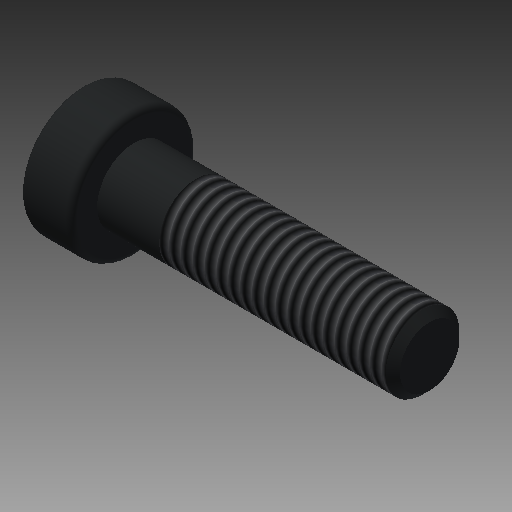
# Autodesk Inventor part: DIN-6912 - M5x20(F)
Saved by Autodesk Inventor 2017 (Build 210142000, 142)
## iProperties
Category: PARTsolutions
Company: FESTO
Created: 2018-05-29
Part Number: DIN-6912 - M5x20(F)
Catalog Web Link: www.cadenas.de
Description: DIN-6912-Hexagon socket head cap screw with centre hole and low head
Vendor: FESTO
Document SubType Name: Modeling
Designer: psAdmin
Manufacturer: FESTO
Mass: 0.545165 g
Surface Area: 5.48093 cm^2
Volume: 0.545165 cm^3
Density: 1 g/cm^3
Material: Generic
Appearance: PSOLRGB-46-51-51
PSOL_IDENT_0: {$CADENAS_DATA\23d-libs\festo\zyl_zubeh\din_6912\din_6912.prj},183 {VTYP=3D},{NB=DIN-6912 - M5x20(F)
PSOL_IDENT_1: },{LINA=DIN-6912 - M5x20(F)},{NN=DIN-6912},{DATE=16.11.2017 11:29:57},{GEOMDATE=16.11.2017 11:29:44}
PSOL_IDENT_2: ,{VERSION=},{LINEID=130},{LINESUBID=-1},{WBVAR=}  {NB=DIN-6912 - M5x20(F)},{LINA=DIN-6912 - M5x20(F)
PSOL_IDENT_3: },{KT=L},{IDNR=},{NENN=M5x20},{D=5.000},{L=20.000},{DK=4.019},{LS=1.800},{LG=4.200},{DK1=8.500},{DH=
PSOL_IDENT_4: 2.500},{K=3.500},{R=0.200},{V=0.400},{S=4.000},{T1=2.000},{T2=4.000},{F=0.600},{DA=5.700},{DW=7.700}
NN: DIN-6912
NT: Hexagon socket head cap screw with centre hole and low head
NB: DIN-6912 - M5x20(F)
NBSYN: DIN-6912 - $NENN.(F)
LINA: DIN-6912 - M5x20(F)
ROWDESC: M5x20
D: 5.000
L: 20.000
DK: 4.019
LS: 1.800
LG: 4.200
DK1: 8.500
DH: 2.500
K: 3.500
R: 0.200
V: 0.400
S: 4.000
T1: 2.000
T2: 4.000
F: 0.600
DA: 5.700
DW: 7.700
SUPPLIER: FESTO
ARTICLENO: DIN-6912 - M5x20(F)
BOMINFO: DIN-6912 - M5x20(F)
CREATOR: CADENAS GmbH
Title: DIN-6912 - M5x20(F)
Author: Cadenas PARTsolutions
Comments: Hexagon socket head cap screw with centre hole and low head
Autodesk Inventor part; units mm, degrees
sketch "Sketch_1" plane through (0, 0, 0) normal (0, 0, 1) x (1, 0, 0)
  line L0 (20, 0) -> (1.75, 0)
  line L1 (1.75, 0) -> (0.5, 1.25)
  line L2 (0.5, 1.25) -> (-0.75, 1.25)
  line L3 (-0.75, 1.25) -> (-1.5, 2)
  line L4 (-1.5, 2) -> (-3.1906, 2)
  line L5 (-3.1906, 2) -> (-3.5, 2.3094)
  line L6 (-3.5, 2.3094) -> (-3.5, 3.85)
  arc A0 (-3.1, 4.25) -> (-3.5, 3.85) centre (-3.1, 3.85) ccw
  line L7 (-3.1, 4.25) -> (-0.4, 4.25)
  arc A1 (0, 3.85) -> (-0.4, 4.25) centre (-0.4, 3.85) ccw
  line L8 (0, 3.85) -> (0, 2.5)
  line L9 (0, 2.5) -> (19.5095, 2.5)
  line L10 (19.5095, 2.5) -> (20, 2.0095)
  line L11 (20, 2.0095) -> (20, 0)
  line L12 (20, 0) -> (1.75, 0)
  constraints: 26 end point, 4 point on circle, 2 centre point
revolve "Revolution1" add sketch "Sketch_1" angle 360 about axis through (20, 0, 0) along (-1, 0, 0)
thread "Thread1" size "M5x0.8" class "6g" standard "ISO Metric profile" length 15.3095
sketch "Sketch_2" plane through (-3.5, 0, 0) normal (1, 0, 0) x (0, 0, -1)
  line L0 (-2, -1.1547) -> (0, -2.3094)
  line L1 (0, -2.3094) -> (2, -1.1547)
  line L2 (2, -1.1547) -> (2, 1.1547)
  line L3 (2, 1.1547) -> (0, 2.3094)
  line L4 (0, 2.3094) -> (-2, 1.1547)
  line L5 (-2, 1.1547) -> (-2, -1.1547)
  constraints: 12 end point
extrude "Extrusion1" cut sketch "Sketch_2" along normal blind 2
ref_plane "MONTAGE_XY" through (0, 0, 0) normal (1, 0, 0) x (0, 0, -1)
ref_plane "MONTAGE_YZ" through (0, 0, 0) normal (0, 0, -1) x (0, 1, 0)
ref_plane "MONTAGE_ZX" through (0, 0, 0) normal (0, 1, 0) x (1, 0, 0)
ref_plane "Schrauben_punkt_XY" through (20, 0, 0) normal (-1, 0, 0) x (0, 0, -1)
ref_plane "Schrauben_punkt_YZ" through (20, 0, 0) normal (0, 0, -1) x (0, -1, 0)
ref_plane "Schrauben_punkt_ZX" through (20, 0, 0) normal (0, -1, 0) x (-1, 0, 0)
body "Solid1"
